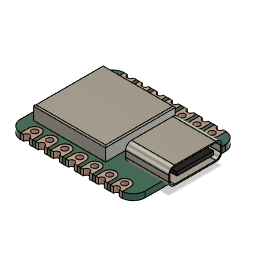
Volume v3 (Autodesk Fusion 360 archive; units mm, degrees)
design "Seeduino XIAO 1"
Autodesk Fusion 360 part; units mm, degrees
sketch "Sketch1" plane through (0, 0, 0) normal (0, 1, 0) x (1, 0, 0) in component "Seeeduino XIAO"
  line L0 (0, 8.8) -> (21.1, 8.8)
  line L1 (21.1, 8.8) -> (21.1, -8.8)
  line L2 (21.1, -8.8) -> (0, -8.8)
  line L3 (0, -8.8) -> (0, 8.8)
  line L4 (22.8, 4.5) -> (15.5, 4.5)
  line L5 (15.5, 4.5) -> (15.5, -4.5)
  line L6 (15.5, -4.5) -> (22.8, -4.5)
  line L7 (22.8, -4.5) -> (22.8, 4.5)
  line L8 (0, 0) -> (15.5, 0) construction
  line L9 (1.3, 5.9) -> (13.5, 5.9)
  line L10 (13.5, 5.9) -> (13.5, -5.9)
  line L11 (13.5, -5.9) -> (1.3, -5.9)
  line L12 (1.3, -5.9) -> (1.3, 5.9)
  circle A0 centre (3, 7.4) radius 0.5
  arc A1 (2.5, 8.8) -> (3.5, 8.8) centre (3, 8.8) ccw
  line L13 (3, 7.4) -> (3, 7.5)
  line L14 (3, 7.5) -> (3, 8.8) construction
  line L15 (4, 8.8) -> (4, 7.4)
  line L16 (2, 8.8) -> (2, 7.4)
  arc A2 (2, 7.4) -> (4, 7.4) centre (3, 7.4) ccw
  line L17 (4, 7.4) -> (2, 7.4) construction
  line L18 (5.54, 7.4) -> (5.54, 7.5)
  line L19 (4.54, 8.8) -> (4.54, 7.4)
  line L20 (5.54, 7.5) -> (5.54, 8.8) construction
  line L21 (6.54, 8.8) -> (6.54, 7.4)
  arc A3 (4.54, 7.4) -> (6.54, 7.4) centre (5.54, 7.4) ccw
  line L22 (6.54, 7.4) -> (4.54, 7.4) construction
  circle A4 centre (5.54, 7.4) radius 0.5
  arc A5 (5.04, 8.8) -> (6.04, 8.8) centre (5.54, 8.8) ccw
  line L23 (8.08, 7.4) -> (8.08, 7.5)
  line L24 (7.08, 8.8) -> (7.08, 7.4)
  line L25 (8.08, 7.5) -> (8.08, 8.8) construction
  line L26 (9.08, 8.8) -> (9.08, 7.4)
  arc A6 (7.08, 7.4) -> (9.08, 7.4) centre (8.08, 7.4) ccw
  line L27 (9.08, 7.4) -> (7.08, 7.4) construction
  circle A7 centre (8.08, 7.4) radius 0.5
  arc A8 (7.58, 8.8) -> (8.58, 8.8) centre (8.08, 8.8) ccw
  line L28 (10.62, 7.4) -> (10.62, 7.5)
  line L29 (9.62, 8.8) -> (9.62, 7.4)
  line L30 (10.62, 7.5) -> (10.62, 8.8) construction
  line L31 (11.62, 8.8) -> (11.62, 7.4)
  arc A9 (9.62, 7.4) -> (11.62, 7.4) centre (10.62, 7.4) ccw
  line L32 (11.62, 7.4) -> (9.62, 7.4) construction
  circle A10 centre (10.62, 7.4) radius 0.5
  arc A11 (10.12, 8.8) -> (11.12, 8.8) centre (10.62, 8.8) ccw
  line L33 (13.16, 7.4) -> (13.16, 7.5)
  line L34 (12.16, 8.8) -> (12.16, 7.4)
  line L35 (13.16, 7.5) -> (13.16, 8.8) construction
  line L36 (14.16, 8.8) -> (14.16, 7.4)
  arc A12 (12.16, 7.4) -> (14.16, 7.4) centre (13.16, 7.4) ccw
  line L37 (14.16, 7.4) -> (12.16, 7.4) construction
  circle A13 centre (13.16, 7.4) radius 0.5
  arc A14 (12.66, 8.8) -> (13.66, 8.8) centre (13.16, 8.8) ccw
  line L38 (15.7, 7.4) -> (15.7, 7.5)
  line L39 (14.7, 8.8) -> (14.7, 7.4)
  line L40 (15.7, 7.5) -> (15.7, 8.8) construction
  line L41 (16.7, 8.8) -> (16.7, 7.4)
  arc A15 (14.7, 7.4) -> (16.7, 7.4) centre (15.7, 7.4) ccw
  line L42 (16.7, 7.4) -> (14.7, 7.4) construction
  circle A16 centre (15.7, 7.4) radius 0.5
  arc A17 (15.2, 8.8) -> (16.2, 8.8) centre (15.7, 8.8) ccw
  line L43 (18.24, 7.4) -> (18.24, 7.5)
  line L44 (17.24, 8.8) -> (17.24, 7.4)
  line L45 (18.24, 7.5) -> (18.24, 8.8) construction
  line L46 (19.24, 8.8) -> (19.24, 7.4)
  arc A18 (17.24, 7.4) -> (19.24, 7.4) centre (18.24, 7.4) ccw
  line L47 (19.24, 7.4) -> (17.24, 7.4) construction
  circle A19 centre (18.24, 7.4) radius 0.5
  arc A20 (17.74, 8.8) -> (18.74, 8.8) centre (18.24, 8.8) ccw
  line L48 (14.16, -8.8) -> (14.16, -7.4)
  arc A21 (19.24, -7.4) -> (17.24, -7.4) centre (18.24, -7.4) ccw
  circle A22 centre (8.08, -7.4) radius 0.5
  line L49 (9.08, -8.8) -> (9.08, -7.4)
  line L50 (7.08, -8.8) -> (7.08, -7.4)
  arc A23 (6.04, -8.8) -> (5.04, -8.8) centre (5.54, -8.8) ccw
  line L51 (5.54, -7.5) -> (5.54, -8.8) construction
  line L52 (3, -7.4) -> (3, -7.5)
  line L53 (6.54, -8.8) -> (6.54, -7.4)
  line L54 (13.16, -7.4) -> (13.16, -7.5)
  line L55 (19.24, -8.8) -> (19.24, -7.4)
  line L56 (10.62, -7.4) -> (10.62, -7.5)
  arc A24 (4, -7.4) -> (2, -7.4) centre (3, -7.4) ccw
  line L57 (11.62, -7.4) -> (9.62, -7.4) construction
  line L58 (16.7, -8.8) -> (16.7, -7.4)
  circle A25 centre (15.7, -7.4) radius 0.5
  circle A26 centre (5.54, -7.4) radius 0.5
  line L59 (15.7, -7.4) -> (15.7, -7.5)
  circle A27 centre (18.24, -7.4) radius 0.5
  line L60 (13.16, -7.5) -> (13.16, -8.8) construction
  line L61 (16.7, -7.4) -> (14.7, -7.4) construction
  arc A28 (16.2, -8.8) -> (15.2, -8.8) centre (15.7, -8.8) ccw
  line L62 (12.16, -8.8) -> (12.16, -7.4)
  circle A29 centre (3, -7.4) radius 0.5
  arc A30 (3.5, -8.8) -> (2.5, -8.8) centre (3, -8.8) ccw
  arc A31 (6.54, -7.4) -> (4.54, -7.4) centre (5.54, -7.4) ccw
  line L63 (18.24, -7.5) -> (18.24, -8.8) construction
  line L64 (10.62, -7.5) -> (10.62, -8.8) construction
  circle A32 centre (10.62, -7.4) radius 0.5
  arc A33 (11.62, -7.4) -> (9.62, -7.4) centre (10.62, -7.4) ccw
  line L65 (5.54, -7.4) -> (5.54, -7.5)
  arc A34 (13.66, -8.8) -> (12.66, -8.8) centre (13.16, -8.8) ccw
  circle A35 centre (13.16, -7.4) radius 0.5
  line L66 (8.08, -7.5) -> (8.08, -8.8) construction
  arc A36 (16.7, -7.4) -> (14.7, -7.4) centre (15.7, -7.4) ccw
  line L67 (8.08, -7.4) -> (8.08, -7.5)
  arc A37 (11.12, -8.8) -> (10.12, -8.8) centre (10.62, -8.8) ccw
  line L68 (2, -8.8) -> (2, -7.4)
  line L69 (17.24, -8.8) -> (17.24, -7.4)
  line L70 (18.24, -7.4) -> (18.24, -7.5)
  line L71 (4.54, -8.8) -> (4.54, -7.4)
  line L72 (9.62, -8.8) -> (9.62, -7.4)
  arc A38 (18.74, -8.8) -> (17.74, -8.8) centre (18.24, -8.8) ccw
  arc A39 (14.16, -7.4) -> (12.16, -7.4) centre (13.16, -7.4) ccw
  line L73 (14.7, -8.8) -> (14.7, -7.4)
  line L74 (19.24, -7.4) -> (17.24, -7.4) construction
  line L75 (4, -7.4) -> (2, -7.4) construction
  arc A40 (8.58, -8.8) -> (7.58, -8.8) centre (8.08, -8.8) ccw
  arc A41 (9.08, -7.4) -> (7.08, -7.4) centre (8.08, -7.4) ccw
  line L76 (3, -7.5) -> (3, -8.8) construction
  line L77 (11.62, -8.8) -> (11.62, -7.4)
  line L78 (14.16, -7.4) -> (12.16, -7.4) construction
  line L79 (15.7, -7.5) -> (15.7, -8.8) construction
  line L80 (4, -8.8) -> (4, -7.4)
  line L81 (9.08, -7.4) -> (7.08, -7.4) construction
  line L82 (6.54, -7.4) -> (4.54, -7.4) construction
  point P0 (1.3, 0)
  dimension "d1" = 21.1
  dimension "d2" = 17.6
  dimension "d3" = 7.3
  dimension "d4" = 9
  dimension "d5" = 1.7
  dimension "d6" = 12.2
  dimension "d7" = 11.8
  dimension "d8" = 1.3
  dimension "d9" = 1.4
  dimension "d10" = 1
  dimension "d11" = 0.5
  dimension "d13" = 2
  dimension "d14" = 2
  dimension "d17" = 2.54
  dimension "d18" = 0
  constraint horizontal L0
  constraint vertical L1
  constraint horizontal L2
  constraint vertical L3
  constraint midpoint L3 L8.start
  constraint coincident L8.start origin
  constraint horizontal L4
  constraint vertical L5
  constraint horizontal L6
  constraint vertical L7
  constraint midpoint L5 L8.end
  constraint horizontal L8
  constraint horizontal L9
  constraint vertical L10
  constraint horizontal L11
  constraint vertical L12
  constraint midpoint L12 P0
  constraint coincident L0 A1.end
  constraint coincident L0 A1.centre
  constraint coincident A0.centre L13.start
  constraint vertical L13
  constraint perpendicular L0 L14
  constraint coincident A1.centre L14.end
  constraint coincident L0 L15.start
  constraint perpendicular L0 L15
  constraint coincident L0 L16.start
  constraint perpendicular L0 L16
  constraint perpendicular L16 L17
  constraint coincident A0.centre L17
  constraint symmetric L8 A0 A29
  constraint symmetric L8 A1.start A30.end
  constraint symmetric L8 A1.end A30.start
  constraint symmetric L8 A1 A30
  constraint symmetric L8 A0.centre L52.start
  constraint symmetric L8 L13.end L52.end
  constraint symmetric L8 A1.centre A30.centre
  constraint symmetric L8 L15.start L80.start
  constraint symmetric L8 L15.end A24.start
  constraint symmetric L8 L16.start L68.start
  constraint symmetric L8 L16.end A24.end
  constraint symmetric L8 A2 A24
  constraint symmetric L8 A5.end A23.start
  constraint symmetric L8 L18.end L51.start
  constraint symmetric L8 L18.start A26.centre
  constraint symmetric L8 A5.start A23.end
  constraint symmetric L8 L20.end A23.centre
  constraint symmetric L8 L21.start L53.start
  constraint symmetric L8 L19.start L71.start
  constraint symmetric L8 L19.end A31.end
  constraint symmetric L8 L21.end L53.end
  constraint symmetric L8 A3 A31
  constraint symmetric L8 A4 A26
  constraint symmetric L8 A5 A23
  constraint symmetric L8 A8.end A40.start
  constraint symmetric L8 L23.end L66.start
  constraint symmetric L8 L23.start A22.centre
  constraint symmetric L8 A8.start A40.end
  constraint symmetric L8 L25.end L66.end
  constraint symmetric L8 L26.start L49.start
  constraint symmetric L8 L24.start L50.start
  constraint symmetric L8 L24.end L50.end
  constraint symmetric L8 L26.end L49.end
  constraint symmetric L8 A6 A41
  constraint symmetric L8 A7 A22
  constraint symmetric L8 A8 A40
  constraint symmetric L8 A11.end A37.start
  constraint symmetric L8 L28.end L56.end
  constraint symmetric L8 L28.start L56.start
  constraint symmetric L8 A11.start A37.end
  constraint symmetric L8 L30.end L64.end
  constraint symmetric L8 L31.start L77.start
  constraint symmetric L8 L29.start L72.start
  constraint symmetric L8 L29.end L57.end
  constraint symmetric L8 L31.end L57.start
  constraint symmetric L8 A9 A33
  constraint symmetric L8 A10 A32
  constraint symmetric L8 A11 A37
  constraint symmetric L8 A14.end A34.start
  constraint symmetric L8 L33.end L54.end
  constraint symmetric L8 L33.start L54.start
  constraint symmetric L8 A14.start A34.end
  constraint symmetric L8 L35.end L60.end
  constraint symmetric L8 L36.start L48.start
  constraint symmetric L8 L34.start L62.start
  constraint symmetric L8 L34.end L62.end
  constraint symmetric L8 L36.end L48.end
  constraint symmetric L8 A12 A39
  constraint symmetric L8 A13 A35
  constraint symmetric L8 A14 A34
  constraint symmetric L8 A17.end A28.start
  constraint symmetric L8 L38.end L59.end
  constraint symmetric L8 L38.start A25.centre
  constraint symmetric L8 A17.start A28.end
  constraint symmetric L8 L40.end A28.centre
  constraint symmetric L8 L41.start L58.start
  constraint symmetric L8 L39.start L73.start
  constraint symmetric L8 L39.end L61.end
  constraint symmetric L8 L41.end L58.end
  constraint symmetric L8 A15 A36
  constraint symmetric L8 A16 A25
  constraint symmetric L8 A17 A28
  constraint symmetric L8 A20.end A38.start
  constraint symmetric L8 L43.end L63.start
  constraint symmetric L8 L43.start A21.centre
  constraint symmetric L8 A20.start A38.end
  constraint symmetric L8 L45.end L63.end
  constraint symmetric L8 L46.start L55.start
  constraint symmetric L8 L44.start L69.start
  constraint symmetric L8 L44.end A21.end
  constraint symmetric L8 L46.end A21.start
  constraint symmetric L8 A18 A21
  constraint symmetric L8 A19 A27
  constraint symmetric L8 A20 A38
  constraint coincident L0 A1.start
  measures "d1" distance of L0.start L0.end
  measures "d2" distance of L0.start L2.end
  measures "d3" distance of L4.start L4.end
  measures "d4" distance of L4.start L6.end
  measures "d5" distance of L1 L7
  measures "d6" distance of L9.start L9.end
  measures "d7" distance of L9.start L11.end
  measures "d8" distance of L3 L12
  measures "d9" distance of L0 A0.centre
  measures "d10" diameter of A0
  measures "d11" radius of A1
  measures "d13" distance of L3 L16
  measures "d14" distance of L15 L16
extrude "Extrude2" add sketch "Sketch1" along normal blind 1 contours L0 L1 L2 L3 L4 L5 L6 L15 L16 A2 L19 L21 A3 L24 L26 A6 L29 L31 A9 L34 L36 A12 L39 L41 A15 L44 L46 A18 L48 A21 L49 L50 L53 L55 A24 L58 L62 A31 A33 A36 L68 L69 L71 L72 A39 L73 A41 L77 L80 | L1 L4 L5 L6 | L9 L10 L11 L12 makes body 1 in component "Seeeduino XIAO"
extrude "Extrude3" add sketch "Sketch1" along normal blind 1 separate body contours L0 A1 L15 L16 A2 | L2 A24 A30 L68 L80 | L0 L19 L21 A3 A5 | L2 A23 L53 A31 L71 | L0 L24 L26 A6 A8 | L2 L49 L50 A40 A41 | L0 L29 L31 A9 A11 | L2 A33 A37 L72 L77 | L0 L34 L36 A12 A14 | L2 L48 L62 A34 A39 | L0 L39 L41 A15 A17 | L2 L58 A28 A36 L73 | L0 L44 L46 A18 A20 | L2 A21 L55 L69 A38 makes body 2 at (13.9644, 0, -7.9606) makes body 3 at (3.8044, 0, -7.9606) makes body 4 at (9.8156, 0, 8.2394) makes body 5 at (17.4356, 0, 8.2394) makes body 6 at (7.2756, 0, 8.2394) makes body 7 at (6.3444, 0, -7.9606) makes body 8 at (14.8956, 0, -8.2394) makes body 9 at (9.8156, 0, -8.2394) makes body 10 at (2.1956, 0, 8.2394) makes body 11 at (12.3556, 0, 8.2394) makes body 12 at (14.8956, 0, 8.2394) makes body 13 at (4.7356, 0, 8.2394) makes body 14 at (7.2756, 0, -7.9606) makes body 15 at (19.0444, 0, -7.9606) in component "Seeeduino XIAO"
fillet "Fillet3" radius 2 4 edges at (0, 0.5, 8.8) (21.1, 0.5, 8.8) (21.1, 0.5, -8.8) (0, 0.5, -8.8) on bodies 1 in component "Seeeduino XIAO"
extrude "Extrude1" add sketch "Sketch1" along normal blind 2.3 from surface at 1 separate body contours L9 L10 L11 L12 makes body 16 in component "Seeeduino XIAO"
extrude "Extrude4" add sketch "Sketch1" along normal blind 3 from surface at 1 separate body contours L1 L4 L6 L7 | L1 L4 L5 L6 makes body 17 in component "Seeeduino XIAO"
fillet "Fillet1" radius 1 4 edges at (19.15, 4, -4.5) (19.15, 1, -4.5) (19.15, 4, 4.5) (19.15, 1, 4.5) on bodies 17 in component "Seeeduino XIAO"
shell "Shell1" thickness 0.2 removed faces 1 at (22.8, 3, -1.1667) on bodies 17 in component "Seeeduino XIAO"
sketch "Sketch1 (1)" plane through (15.7, 0, 0) normal (1, 0, 0) x (0, 0, -1) in component "Seeeduino XIAO"
  arc A0 (-4.3, 2) -> (-3.5, 1.2) centre (-3.5, 2) ccw
  line L0 (-3.5, 1.2) -> (3.5, 1.2)
  arc A1 (3.5, 1.2) -> (4.3, 2) centre (3.5, 2) ccw
  line L1 (4.3, 2) -> (4.3, 3)
  arc A2 (4.3, 3) -> (3.5, 3.8) centre (3.5, 3) ccw
  line L2 (3.5, 3.8) -> (-3.5, 3.8)
  arc A3 (-3.5, 3.8) -> (-4.3, 3) centre (-3.5, 3) ccw
  line L3 (-4.3, 3) -> (-4.3, 2)
  line L4 (-3.1, 2.8) -> (3.1, 2.8)
  line L5 (3.1, 2.8) -> (3.1, 2.2)
  line L6 (3.1, 2.2) -> (-3.1, 2.2)
  line L7 (-3.1, 2.2) -> (-3.1, 2.8)
  line L8 (0, 1.2) -> (0, 2.2) construction
  line L9 (-3.1, 2.5) -> (-4.3, 2.5) construction
  dimension "d35" = 6.2
  dimension "d36" = 0.6
  constraint horizontal L4
  constraint vertical L5
  constraint horizontal L6
  constraint vertical L7
  constraint midpoint L0 L8.start
  constraint midpoint L6 L8.end
  constraint perpendicular L6 L8
  constraint midpoint L7 L9.start
  constraint midpoint L3 L9.end
  constraint horizontal L9
  measures "d35" distance of L4.start L4.end
  measures "d36" distance of L4.start L6.end
extrude "Extrude5" add sketch "Sketch1 (1)" along normal blind 7.1 separate body contours L4 L5 L6 L7 makes body 18 in component "Seeeduino XIAO"
fillet "Fillet2" radius 0.2 4 edges at (7.4, 3.3, 5.9) (13.5, 3.3, 0) (7.4, 3.3, -5.9) (1.3, 3.3, 0) on bodies 16 in component "Seeeduino XIAO"
component "Seeeduino XIAO" placed x (1, 0, 0) y (0, 1, 0) z (0, 0, 1) at (0, 0, 0)
